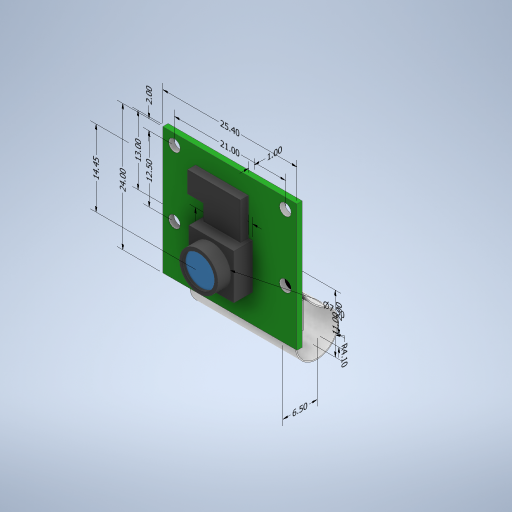
# Autodesk Inventor part: cam
Saved by Autodesk Inventor 2024.1 (Build 281209000, 209)
## iProperties
Created: 2025-01-10
Part Number: cam
Material: 一般
Document SubType Name: Modeling
Designer: hibik
Density: 1 g/cm^3
Appearance: 既定
Author: hibik
Autodesk Inventor part; units mm, degrees
ref_plane "YZ Plane" through (0, 0, 0) normal (1, 0, 0) x (0, 1, 0)
ref_plane "XZ Plane" through (0, 0, 0) normal (0, 1, 0) x (-1, 0, 0)
ref_plane "XY Plane" through (0, 0, 0) normal (0, 0, 1) x (1, 0, 0)
sketch "スケッチ1" plane through (0, 0, 0) normal (0, 0, 1) x (1, 0, 0)
  line L0 (-12.7, 14.45) -> (12.7, 14.45)
  line L1 (12.7, 14.45) -> (12.7, -9.55)
  line L2 (12.7, -9.55) -> (-12.7, -9.55)
  line L3 (-12.7, -9.55) -> (-12.7, 14.45)
  line L4 (-12.7, 14.45) -> (12.7, -9.55) construction
  line L5 (12.7, 14.45) -> (-12.7, -9.55) construction
  point P0 (0, 0)
  point P1 (0, 2.45)
  dimension "d0" = 25.4
  dimension "d1" = 24
  dimension "d2" = 14.45
  constraints: 12 end point, 2 midpoint, 2 parallel, 1 horizontal, 1 perpendicular, 1 vertical alignment
  measures "d0" distance of L1.end L2.end
  measures "d1" distance of L0.end L1.end
  measures "d2" distance from line of point (0, 0) L0
extrude "押し出し1" add sketch "スケッチ1" along normal blind 1
sketch "スケッチ2" plane through (0, 0, 1) normal (0, 0, 1) x (1, 0, 0)
  line L0 (4.25, 4.25) -> (-4.25, 4.25)
  line L1 (-4.25, 4.25) -> (-4.25, -4.25)
  line L2 (-4.25, -4.25) -> (4.25, -4.25)
  line L3 (4.25, -4.25) -> (4.25, 4.25)
  line L4 (4.25, 4.25) -> (-4.25, -4.25) construction
  line L5 (-4.25, 4.25) -> (4.25, -4.25) construction
  point P0 (0, 0)
  dimension "d5" = 8.5
  constraints: 12 end point, 2 midpoint, 2 parallel, 2 perpendicular, 1 horizontal
  measures "d5" distance of L2.end L1.end
extrude "押し出し2" add sketch "スケッチ2" along normal blind 3.5
sketch "スケッチ3" plane through (0, 0, 4.5) normal (0, 0, 1) x (1, 0, 0)
  circle A0 centre (0, 0) radius 3.65
  dimension "d8" = 7.3
  constraints: 1 centre point, 1 coincident
  measures "d8" diameter of A0
extrude "押し出し3" add sketch "スケッチ3" along normal blind 2.4
sketch "スケッチ4" plane through (0, 0, 6.9) normal (0, 0, 1) x (1, 0, 0)
  circle A0 centre (0, 0) radius 3
  dimension "d11" = 6
  constraints: 1 centre point, 1 coincident
  measures "d11" diameter of A0
extrude "押し出し4" cut sketch "スケッチ4" against normal blind 0.5
sketch "スケッチ5" plane through (0, 0, 1) normal (0, 0, 1) x (1, 0, 0)
  line L0 (10.5, -0.05) -> (-10.5, -0.05) construction
  line L1 (-10.5, -0.05) -> (-10.5, 12.45) construction
  line L2 (-10.5, 12.45) -> (10.5, 12.45) construction
  line L3 (10.5, 12.45) -> (10.5, -0.05) construction
  line L4 (10.5, -0.05) -> (-10.5, 12.45) construction
  line L5 (-10.5, -0.05) -> (10.5, 12.45) construction
  line L6 (12.7, 14.45) -> (-12.7, 14.45) projected
  circle A0 centre (-10.5, 12.45) radius 1.1
  circle A1 centre (10.5, 12.45) radius 1.1
  circle A2 centre (-10.5, -0.05) radius 1.1
  circle A3 centre (10.5, -0.05) radius 1.1
  point P0 (0, 0)
  point P1 (0, 6.2)
  dimension "d14" = 21
  dimension "d15" = 12.5
  dimension "d16" = 2
  dimension "d17" = 2.2
  constraints: 12 end point, 4 centre point, 4 coincident, 3 equal radius, 2 midpoint, 2 parallel, 1 horizontal, 1 perpendicular, 1 vertical alignment
  measures "d14" distance of L1.end L2.end
  measures "d15" distance of L0.end L1.end
  measures "d16" distance between parallel lines of L6 L2
  measures "d17" diameter of A0
extrude "押し出し5" cut sketch "スケッチ5" against normal through all
sketch "スケッチ6" plane through (0, 0, 0) normal (0, 0, -1) x (-1, 0, 0)
  line L0 (10, -4.55) -> (-10, -4.55)
  line L1 (-10, -4.55) -> (-10, -9.55)
  line L2 (-10, -9.55) -> (10, -9.55)
  line L3 (10, -9.55) -> (10, -4.55)
  line L4 (10, -4.55) -> (-10, -9.55) construction
  line L5 (-10, -4.55) -> (10, -9.55) construction
  line L6 (12.7, -9.55) -> (-12.7, -9.55) projected
  point P0 (0, 0)
  point P1 (0, -7.05)
  dimension "d20" = 20
  dimension "d21" = 5
  constraints: 12 end point, 2 midpoint, 2 parallel, 1 collinear, 1 horizontal, 1 perpendicular, 1 vertical alignment
  measures "d20" distance of L1.end L2.end
  measures "d21" distance of L2.end L0.start
extrude "押し出し6" add sketch "スケッチ6" along normal blind 3
sketch "スケッチ7" plane through (0, 0, 0) normal (0, 0, -1) x (-1, 0, 0)
  line L0 (8.5, 1.2) -> (-8.5, 1.2)
  line L1 (-8.5, 1.2) -> (-8.5, 11.2)
  line L2 (-8.5, 11.2) -> (8.5, 11.2)
  line L3 (8.5, 11.2) -> (8.5, 1.2)
  line L4 (8.5, 1.2) -> (-8.5, 11.2) construction
  line L5 (-8.5, 1.2) -> (8.5, 11.2) construction
  circle A0 centre (-10.5, 12.45) radius 1.1 projected
  circle A1 centre (-10.5, -0.05) radius 1.1 projected
  point P0 (0, 0)
  point P1 (0, 6.2)
  dimension "d24" = 17
  dimension "d25" = 10
  dimension "d26" = 6.25
  dimension "d27" = 6.25
  constraints: 12 end point, 2 midpoint, 2 parallel, 1 horizontal, 1 perpendicular, 1 vertical alignment
  measures "d24" distance of L1.end L2.end
  measures "d25" distance of L0.end L1.end
  measures "d26" vertical distance of A0.centre point (0, 6.2)
  measures "d27" vertical distance of A1.centre point (0, 6.2)
extrude "押し出し7" add sketch "スケッチ7" along normal blind 1 contours L0 L1 L2 L3
sketch "スケッチ8" plane through (10, -9.55, 0) normal (1, 0, 0) x (0, 0, -1)
  line L0 (1.6, -2) -> (1.4, -2) construction
  line L1 (1.4, -2) -> (1.4, 0)
  line L2 (1.4, 0) -> (1.6, 0)
  line L3 (1.6, 0) -> (1.6, -2)
  line L4 (1.6, -2) -> (1.4, 0) construction
  line L5 (1.4, -2) -> (1.6, 0) construction
  line L6 (0, 0) -> (3, 0) projected
  circle A0 centre (5.5, -2) radius 4 construction
  line L7 (1.5, 0) -> (1.5, -2) construction
  circle A1 centre (5.5, -2) radius 4.1
  circle A2 centre (5.5, -2) radius 3.9
  arc A3 (1.4, 11) -> (7.2575, 1.4815) centre (12.0625, 11) ccw
  line L8 (1.4, 0) -> (1.4, 9.037) construction
  line L9 (1.6, 0) -> (1.6, 10.1272) construction
  arc A4 (1.6, 11) -> (7.3476, 1.6601) centre (12.0625, 11) ccw
  line L10 (1.4, 11) -> (1.6, 11)
  point P0 (0, 9.55)
  point P1 (1.5, -1)
  dimension "d30" = 0.2
  dimension "d31" = 2
  dimension "d32" = 8
  dimension "d33" = 11
  constraints: 20 end point, 8 point on circle, 5 centre point, 5 tangent, 4 midpoint, 2 coincident, 2 horizontal, 2 horizontal alignment, 2 parallel, 2 point on line, 2 vertical, 1 collinear, 1 perpendicular, 1 vertical alignment
  measures "d30" distance of L1.end L2.end
  measures "d31" distance of L0.end L1.end
  measures "d32" diameter of A0
  measures "d33" distance from line of L6 L10.start
extrude "押し出し8" add sketch "スケッチ8" against normal up to surface (20 mm away) contours A1 L3 A2 A3 | L1 L2 L3 A1 | A1 A3 L10 A4
sketch "スケッチ9" plane through (0, 0, 1) normal (0, 0, 1) x (1, 0, 0)
  line L0 (-3.5, 11.25) -> (3.5, 11.25)
  line L1 (3.5, 11.25) -> (3.5, 4.25)
  line L2 (3.5, 4.25) -> (-3.5, 4.25)
  line L3 (-3.5, 4.25) -> (-3.5, 11.25)
  line L4 (-3.5, 11.25) -> (3.5, 4.25) construction
  line L5 (3.5, 11.25) -> (-3.5, 4.25) construction
  line L6 (-4.25, 4.25) -> (4.25, 4.25) projected
  line L7 (3.5, 11.25) -> (-6.5, 11.25)
  line L8 (-6.5, 11.25) -> (-6.5, 7.25)
  line L9 (-6.5, 7.25) -> (3.5, 7.25)
  line L10 (3.5, 7.25) -> (3.5, 11.25)
  point P0 (0, 0)
  point P1 (0, 7.75)
  point P2 (-3.5, 7.25)
  dimension "d65" = 7
  dimension "d66" = 7
  dimension "d67" = 10
  dimension "d68" = 4
  constraints: 20 end point, 4 parallel, 2 horizontal, 2 midpoint, 2 perpendicular, 1 collinear, 1 vertical alignment
  measures "d65" distance of L1.end L2.end
  measures "d66" distance of L0.end L1.end
  measures "d67" distance of L9.end L8.end
  measures "d68" distance of L8.end L7.end
extrude "押し出し9" add sketch "スケッチ9" along normal blind 1.5
equation "\"d26\" = d27"
